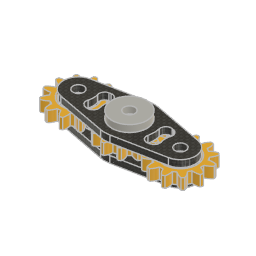
Gear fidget spinner thingy (Autodesk Fusion 360 design; units mm, degrees)
Autodesk Fusion 360 part; units mm, degrees
sketch "Sketch1" plane through (0, 0, 0) normal (0, 0, 1) x (1, 0, 0)
  circle A0 centre (0, 0) radius 12
  line L0 (0, 0) -> (-37, 0) construction
  line L1 (0, 0) -> (37, 0) construction
  line L2 (-37, 0) -> (-37, 25) construction
  line L3 (-37, 0) -> (-37, -25) construction
  circle A1 centre (37, 0) radius 4
  circle A2 centre (-37, 0) radius 4
  line L4 (-3.4054, 17.6749) -> (-39.0811, 10.8013)
  line L5 (3.4054, 17.6749) -> (39.0811, 10.8013)
  line L6 (-3.4054, -17.6749) -> (-39.0811, -10.8013)
  arc A3 (-37, 11) -> (-37, -11) centre (-37, 0) ccw
  arc A4 (38.8507, -10.8432) -> (39.0811, 10.8013) centre (37, 0) ccw
  arc A5 (3.4054, 17.6749) -> (-3.4054, 17.6749) centre (0, 0) ccw
  arc A6 (-3.4054, -17.6749) -> (3.4054, -17.6749) centre (0, 0) ccw
  line L7 (18, 0) -> (26, 0) construction
  line L8 (18, 0) -> (22, 0) construction
  line L9 (-26, 0) -> (-18, 0) construction
  line L10 (-26, 0) -> (-22, 0) construction
  line L11 (-22, 0) -> (-22, 14) construction
  line L12 (-22, 14) -> (-22, -14.0923) construction
  line L13 (22, 0) -> (22, 14.0923) construction
  line L14 (22, 0) -> (22, -14.0923) construction
  line L15 (24.9994, 13.5145) -> (24.0534, 8.6047) construction
  line L16 (38.8512, -10.8456) -> (37.9053, -5.9359) construction
  line L17 (-22, -14.0923) -> (-21.9955, -14.0932) construction
  line L18 (-22, -14.0923) -> (-21.0541, -9.1826) construction
  line L19 (22.1718, 8.9673) -> (23.5375, 8.7041)
  line L20 (23.5375, -8.7041) -> (22.1718, -8.9673)
  line L21 (-22.1718, 8.9673) -> (-23.5375, 8.7041)
  line L22 (39.0811, -10.8013) -> (37, -11.2023)
  line L23 (38.8512, -10.8456) -> (3.4054, -17.6749)
  arc A7 (26.5726, 3.5027) -> (26.5726, -3.5027) centre (37, 0) ccw
  arc A8 (39.0811, -10.8013) -> (39.0811, 10.8013) centre (37, 0) ccw
  arc A9 (17.5214, -4.1232) -> (17.5214, 4.1232) centre (0, 0) ccw
  arc A10 (3.4054, 17.6749) -> (-3.4054, 17.6749) centre (0, 0) ccw
  arc A11 (-17.5214, 4.1232) -> (-17.5214, -4.1232) centre (0, 0) ccw
  arc A12 (-3.4054, -17.6749) -> (3.4054, -17.6749) centre (0, 0) ccw
  line L24 (-22.1718, -8.9673) -> (-23.5375, -8.7041)
  arc A13 (-26.5726, -3.5027) -> (-26.5726, 3.5027) centre (-37, 0) ccw
  arc A14 (-37, 11) -> (-37, -11) centre (-37, 0) ccw
  arc A15 (-17.5214, 4.1232) -> (-22.1718, 8.9673) centre (-21.415, 5.0395) ccw
  arc A16 (-23.5375, 8.7041) -> (-26.5726, 3.5027) centre (-22.7808, 4.7764) ccw
  arc A17 (-26.5726, -3.5027) -> (-23.5375, -8.7041) centre (-22.7808, -4.7764) ccw
  arc A18 (-22.1718, -8.9673) -> (-17.5214, -4.1232) centre (-21.415, -5.0395) ccw
  arc A19 (22.1718, 8.9673) -> (17.5214, 4.1232) centre (21.415, 5.0395) ccw
  arc A20 (26.5726, 3.5027) -> (23.5375, 8.7041) centre (22.7808, 4.7764) ccw
  arc A21 (23.5375, -8.7041) -> (26.5726, -3.5027) centre (22.7808, -4.7764) ccw
  arc A22 (17.5214, -4.1232) -> (22.1718, -8.9673) centre (21.415, -5.0395) ccw
  dimension "d1" = 24
  dimension "d2" = 36
  dimension "d3" = 37
  dimension "d4" = 37
  dimension "d5" = 8
  dimension "d6" = 22
  dimension "d7" = 8
  dimension "d8" = 22
  dimension "d9" = 36
  dimension "d10" = 22
  dimension "d11" = 22
  dimension "d12" = 5
  dimension "d13" = 5
  dimension "d14" = 5
  dimension "d17" = 4
  dimension "d18" = 4
  constraint coincident A0.centre L0.start
  constraint concentric A0 A5
  constraint horizontal L0
  constraint parallel L0 L1
  constraint perpendicular L0 L2
  constraint perpendicular L0 L3
  constraint coincident L1.end A1.centre
  constraint concentric A1 A4
  constraint coincident L0.end L2.start
  constraint concentric A2 A3
  constraint coincident L4.end A3
  constraint tangent L4 A3
  constraint tangent L4 A5
  constraint tangent L5 A4
  constraint tangent L5 A5
  constraint coincident L22.start A4
  constraint tangent A5 L22
  constraint coincident L6.start A5
  constraint coincident L6.end A3
  constraint tangent L6 A3
  constraint tangent L6 A5
  constraint tangent A4 L22
  constraint coincident L2 A3.start
  constraint coincident L3 A3.end
  constraint concentric A5 A6
  constraint concentric A0 A9
  constraint concentric A1 A7
  constraint coincident L1 L7.start
  constraint coincident L7.start A9
  constraint coincident L7.end A7
  constraint coincident L1 L7.end
  constraint midpoint L7 L8.end
  constraint concentric A2 A13
  constraint coincident L9.start A13
  constraint coincident L0 L9.start
  constraint coincident L0 L9.end
  constraint coincident L9.end A9
  constraint midpoint L9 L10.end
  constraint perpendicular L10 L11
  constraint coincident L6 L12.end
  constraint perpendicular L10 L12
  constraint coincident L5 L13.end
  constraint perpendicular L7 L13
  constraint coincident L14.end L22
  constraint perpendicular L1 L14
  constraint coincident L5 L15.start
  constraint perpendicular L5 L15
  constraint coincident L16.start L22
  constraint perpendicular L16 L22
  constraint coincident L6 L17.end
  constraint perpendicular L17 L18
  constraint collinear L22 L23
  constraint concentric A7 A8
  constraint concentric A9 A10
  constraint concentric A10 A11
  constraint concentric A11 A12
  constraint concentric A13 A14
  constraint tangent A11 A15
  constraint tangent L21 A15
  constraint tangent L21 A16
  constraint tangent A13 A16
  constraint equal A15 A16
  constraint tangent A13 A17
  constraint tangent L24 A17
  constraint equal A15 A17
  constraint tangent L24 A18
  constraint tangent A11 A18
  constraint equal A15 A18
  constraint tangent A9 A19
  constraint tangent L19 A19
  constraint tangent L19 A20
  constraint tangent A7 A20
  constraint equal A19 A20
  constraint tangent A7 A21
  constraint tangent L20 A21
  constraint equal A19 A21
  constraint tangent L20 A22
  constraint tangent A9 A22
  constraint equal A19 A22
  constraint tangent L23 A8
  constraint coincident L16 A4.start
  measures "d1" diameter of A0
  measures "d2" diameter of A5
  measures "d3" distance of A0.centre L0.end
  measures "d4" distance of A0.centre L1.end
  measures "d5" diameter of A1
  measures "d6" diameter of A4
  measures "d7" diameter of A2
  measures "d8" diameter of A3
  measures "d9" diameter of A9
  measures "d10" diameter of A7
  measures "d11" diameter of A13
  measures "d12" distance of L15.start L15.end
  measures "d13" distance of L16.start L16.end
  measures "d14" distance of L12.end L18.end
  measures "d17" radius of A15
  measures "d18" radius of A19
extrude "Extrude1" add sketch "Sketch1" along normal blind 5 makes body 1
copy_body "CopyPasteBodies1" bodies 1 makes body 2
move_body "Move1" bodies 2 to x (1, 0, 0) y (0, 1, 0) z (0, 0, 1) at (0, 0, 13)
sketch "Sketch2" plane through (0, 0, 0) normal (0, 0, 1) x (1, 0, 0)
  circle A0 centre (0, 50) radius 12
  line L0 (0, 50) -> (0, 50.4627) construction
  line L1 (0, 70) -> (-1, 70)
  line L2 (0, 70) -> (1, 70)
  line L3 (-10, 67.3205) -> (-9.134, 67.8205)
  line L4 (-10, 67.3205) -> (-10.866, 66.8205)
  line L5 (-17.7256, 59.2984) -> (-16.8205, 60.866)
  line L6 (-17.3205, 60) -> (-17.8205, 59.134)
  line L7 (-20, 50) -> (-20, 51)
  line L8 (-20, 50) -> (-20, 49)
  line L9 (-17.3205, 40) -> (-17.8205, 40.866)
  line L10 (-17.3205, 40) -> (-16.8205, 39.134)
  line L11 (-10, 32.6795) -> (-10.866, 33.1795)
  line L12 (-10, 32.6795) -> (-9.134, 32.1795)
  line L13 (0, 30) -> (-1, 30)
  line L14 (0, 30) -> (1, 30)
  line L15 (10, 32.6795) -> (9.134, 32.1795)
  line L16 (10, 32.6795) -> (10.866, 33.1795)
  line L17 (17.3205, 40) -> (16.8205, 39.134)
  line L18 (17.3205, 40) -> (17.8205, 40.866)
  line L19 (20, 50) -> (20, 49)
  line L20 (20, 50) -> (20, 51)
  line L21 (17.3205, 60) -> (17.8205, 59.134)
  line L22 (17.3205, 60) -> (16.8205, 60.866)
  line L23 (10, 67.3205) -> (10.866, 66.8205)
  line L24 (10, 67.3205) -> (9.134, 67.8205)
  arc A1 (-17.7256, 59.2984) -> (-17.6928, 58.9935) centre (-17.5004, 59.1684) ccw
  line L25 (0, 0) -> (0, 30)
  line L26 (0, 70) -> (0, 75)
  arc A2 (-1, 70) -> (-2.675, 64.7596) centre (7.824, 64.2917) ccw
  arc A3 (2.675, 64.7596) -> (1, 70) centre (-9.0903, 63.8869) ccw
  arc A4 (-5.0632, 64.1196) -> (-9.134, 67.8205) centre (-14.8159, 57.4813) ccw
  arc A5 (-10.866, 66.8205) -> (-9.6964, 61.4446) centre (-0.37, 66.289) ccw
  line L27 (-10, 67.3205) -> (-9.134, 67.8205)
  line L28 (-10, 67.3205) -> (-10.866, 66.8205)
  arc A6 (-11.4446, 59.6964) -> (-16.8205, 60.866) centre (-16.5716, 49.0711) ccw
  arc A7 (-17.8205, 59.134) -> (-14.1196, 55.0632) centre (-8.4649, 63.9216) ccw
  line L29 (-17.3205, 60) -> (-16.8205, 60.866)
  line L30 (-17.3205, 60) -> (-17.8205, 59.134)
  arc A8 (-14.7596, 52.675) -> (-20, 51) centre (-13.8869, 40.9097) ccw
  arc A9 (-20, 49) -> (-14.7596, 47.325) centre (-14.2917, 57.824) ccw
  line L31 (-20, 50) -> (-20, 51)
  line L32 (-20, 50) -> (-20, 49)
  arc A10 (-14.1196, 44.9368) -> (-17.8205, 40.866) centre (-7.4813, 35.1841) ccw
  arc A11 (-16.8205, 39.134) -> (-11.4446, 40.3036) centre (-16.289, 49.63) ccw
  line L33 (-17.3205, 40) -> (-17.8205, 40.866)
  line L34 (-17.3205, 40) -> (-16.8205, 39.134)
  arc A12 (-9.6964, 38.5554) -> (-10.866, 33.1795) centre (0.9289, 33.4284) ccw
  arc A13 (-9.134, 32.1795) -> (-5.0632, 35.8804) centre (-13.9216, 41.5351) ccw
  line L35 (-10, 32.6795) -> (-10.866, 33.1795)
  line L36 (-10, 32.6795) -> (-9.134, 32.1795)
  arc A14 (-2.675, 35.2404) -> (-1, 30) centre (9.0903, 36.1131) ccw
  arc A15 (1, 30) -> (2.675, 35.2404) centre (-7.824, 35.7083) ccw
  line L37 (0, 30) -> (-1, 30)
  line L38 (0, 30) -> (1, 30)
  arc A16 (5.0632, 35.8804) -> (9.134, 32.1795) centre (14.8159, 42.5187) ccw
  arc A17 (10.866, 33.1795) -> (9.6964, 38.5554) centre (0.37, 33.711) ccw
  line L39 (10, 32.6795) -> (9.134, 32.1795)
  line L40 (10, 32.6795) -> (10.866, 33.1795)
  arc A18 (11.4446, 40.3036) -> (16.8205, 39.134) centre (16.5716, 50.9289) ccw
  arc A19 (17.8205, 40.866) -> (14.1196, 44.9368) centre (8.4649, 36.0784) ccw
  line L41 (17.3205, 40) -> (16.8205, 39.134)
  line L42 (17.3205, 40) -> (17.8205, 40.866)
  arc A20 (14.7596, 47.325) -> (20, 49) centre (13.8869, 59.0903) ccw
  arc A21 (20, 51) -> (14.7596, 52.675) centre (14.2917, 42.176) ccw
  line L43 (20, 50) -> (20, 49)
  line L44 (20, 50) -> (20, 51)
  arc A22 (14.1196, 55.0632) -> (17.8205, 59.134) centre (7.4813, 64.8159) ccw
  arc A23 (16.8205, 60.866) -> (11.4446, 59.6964) centre (16.289, 50.37) ccw
  line L45 (17.3205, 60) -> (17.8205, 59.134)
  line L46 (17.3205, 60) -> (16.8205, 60.866)
  arc A24 (9.6964, 61.4446) -> (10.866, 66.8205) centre (-0.9289, 66.5716) ccw
  arc A25 (9.134, 67.8205) -> (5.0632, 64.1196) centre (13.9216, 58.4649) ccw
  line L47 (10, 67.3205) -> (10.866, 66.8205)
  line L48 (10, 67.3205) -> (9.134, 67.8205)
  arc A26 (-2.675, 64.7596) -> (-5.0632, 64.1196) centre (0, 50) ccw
  arc A27 (5.0632, 64.1196) -> (2.675, 64.7596) centre (0, 50) ccw
  arc A28 (-9.6964, 61.4446) -> (-11.4446, 59.6964) centre (0, 50) ccw
  arc A29 (-14.1196, 55.0632) -> (-14.7596, 52.675) centre (0, 50) ccw
  arc A30 (2.675, 35.2404) -> (5.0632, 35.8804) centre (0, 50) ccw
  arc A31 (-5.0632, 35.8804) -> (-2.675, 35.2404) centre (0, 50) ccw
  arc A32 (-14.7596, 47.325) -> (-14.1196, 44.9368) centre (0, 50) ccw
  arc A33 (-11.4446, 40.3036) -> (-9.6964, 38.5554) centre (0, 50) ccw
  arc A34 (11.4446, 59.6964) -> (9.6964, 61.4446) centre (0, 50) ccw
  arc A35 (14.7596, 52.675) -> (14.1196, 55.0632) centre (0, 50) ccw
  arc A36 (9.6964, 38.5554) -> (11.4446, 40.3036) centre (0, 50) ccw
  arc A37 (14.1196, 44.9368) -> (14.7596, 47.325) centre (0, 50) ccw
  dimension "d21" = 24
  dimension "d22" = 30
  dimension "d25" = 20
  dimension "d26" = 1
  dimension "d27" = 1
  dimension "d30" = 0.26
  dimension "d32" = 360
  constraint coincident L25.start origin
  constraint vertical L25
  constraint coincident A0.centre L25
  constraint concentric A0 A26
  constraint coincident A0.centre L0.start
  constraint coincident L0.end L25
  constraint perpendicular L1 L25
  constraint perpendicular L2 L25
  constraint coincident L6.start L5
  constraint tangent L5 A1
  constraint collinear L25 L26
  constraint concentric A26 A28
  constraint concentric A27 A28
  constraint concentric A28 A32
  constraint concentric A28 A29
  constraint concentric A32 A36
  constraint concentric A30 A32
  constraint concentric A31 A32
  constraint concentric A32 A33
  constraint concentric A34 A36
  constraint concentric A35 A36
  constraint concentric A36 A37
  measures "d21" diameter of A0
  measures "d22" diameter of A26
  measures "d25" distance of A0.centre L1.start
  measures "d26" distance of L1.start L1.end
  measures "d27" distance of L1.start L2.end
  measures "d30" radius of A1
extrude "Extrude2" add sketch "Sketch2" along normal blind 8 separate body makes body 3
sketch "Sketch3" plane through (0, 0, 0) normal (0, 0, 1) x (1, 0, 0)
  circle A0 centre (0, 125) radius 12
  line L0 (-1, 145) -> (1, 145) construction
  line L1 (0, 145) -> (-1, 145)
  line L2 (0, 145) -> (1, 145)
  arc A1 (-1, 145) -> (-2.675, 139.7596) centre (8.0445, 139.2212) ccw
  arc A2 (2.675, 139.7596) -> (1, 145) centre (-8.4873, 139.0797) ccw
  line L3 (2.675, 145) -> (2.675, 145.0175) construction
  line L4 (2.675, 145.0175) -> (2.675, 145) construction
  line L5 (-1, 145) -> (1, 145)
  arc A3 (-5.0632, 139.1196) -> (-9.134, 142.8205) centre (-14.3901, 132.9497) ccw
  arc A4 (-10.866, 141.8205) -> (-9.6964, 136.4446) centre (-0.1439, 141.3382) ccw
  line L6 (-10.866, 141.8205) -> (-9.134, 142.8205) construction
  arc A5 (-11.4446, 134.6964) -> (-16.8205, 135.866) centre (-16.437, 124.6896) ccw
  arc A6 (-17.8205, 134.134) -> (-14.1196, 130.0632) centre (-8.2937, 139.0773) ccw
  line L7 (-17.8205, 134.134) -> (-16.8205, 135.866) construction
  arc A7 (-14.7596, 127.675) -> (-20, 126) centre (-14.0797, 116.5127) ccw
  arc A8 (-20, 124) -> (-14.7596, 122.325) centre (-14.2212, 133.0445) ccw
  line L8 (-20, 124) -> (-20, 126) construction
  arc A9 (-14.1196, 119.9368) -> (-17.8205, 115.866) centre (-7.9497, 110.6099) ccw
  arc A10 (-16.8205, 114.134) -> (-11.4446, 115.3036) centre (-16.3382, 124.8561) ccw
  line L9 (-16.8205, 114.134) -> (-17.8205, 115.866) construction
  arc A11 (-9.6964, 113.5554) -> (-10.866, 108.1795) centre (0.3104, 108.563) ccw
  arc A12 (-9.134, 107.1795) -> (-5.0632, 110.8804) centre (-14.0773, 116.7063) ccw
  line L10 (-9.134, 107.1795) -> (-10.866, 108.1795) construction
  arc A13 (-2.675, 110.2404) -> (-1, 105) centre (8.4873, 110.9203) ccw
  arc A14 (1, 105) -> (2.675, 110.2404) centre (-8.0445, 110.7788) ccw
  line L11 (1, 105) -> (-1, 105) construction
  arc A15 (5.0632, 110.8804) -> (9.134, 107.1795) centre (14.3901, 117.0503) ccw
  arc A16 (10.866, 108.1795) -> (9.6964, 113.5554) centre (0.1439, 108.6618) ccw
  line L12 (10.866, 108.1795) -> (9.134, 107.1795) construction
  arc A17 (11.4446, 115.3036) -> (16.8205, 114.134) centre (16.437, 125.3104) ccw
  arc A18 (17.8205, 115.866) -> (14.1196, 119.9368) centre (8.2937, 110.9227) ccw
  line L13 (17.8205, 115.866) -> (16.8205, 114.134) construction
  arc A19 (14.7596, 122.325) -> (20, 124) centre (14.0797, 133.4873) ccw
  arc A20 (20, 126) -> (14.7596, 127.675) centre (14.2212, 116.9555) ccw
  line L14 (20, 126) -> (20, 124) construction
  arc A21 (14.1196, 130.0632) -> (17.8205, 134.134) centre (7.9497, 139.3901) ccw
  arc A22 (16.8205, 135.866) -> (11.4446, 134.6964) centre (16.3382, 125.1439) ccw
  line L15 (16.8205, 135.866) -> (17.8205, 134.134) construction
  arc A23 (9.6964, 136.4446) -> (10.866, 141.8205) centre (-0.3104, 141.437) ccw
  arc A24 (9.134, 142.8205) -> (5.0632, 139.1196) centre (14.0773, 133.2937) ccw
  line L16 (9.134, 142.8205) -> (10.866, 141.8205) construction
  arc A25 (-9.6964, 136.4446) -> (-11.4446, 134.6964) centre (0, 125) ccw
  arc A26 (-14.1196, 130.0632) -> (-14.7596, 127.675) centre (0, 125) ccw
  arc A27 (-14.7596, 122.325) -> (-14.1196, 119.9368) centre (0, 125) ccw
  arc A28 (-11.4446, 115.3036) -> (-9.6964, 113.5554) centre (0, 125) ccw
  arc A29 (-5.0632, 110.8804) -> (-2.675, 110.2404) centre (0, 125) ccw
  arc A30 (2.675, 110.2404) -> (5.0632, 110.8804) centre (0, 125) ccw
  arc A31 (9.6964, 113.5554) -> (11.4446, 115.3036) centre (0, 125) ccw
  arc A32 (14.1196, 119.9368) -> (14.7596, 122.325) centre (0, 125) ccw
  arc A33 (14.7596, 127.675) -> (14.1196, 130.0632) centre (0, 125) ccw
  arc A34 (11.4446, 134.6964) -> (9.6964, 136.4446) centre (0, 125) ccw
  arc A35 (5.0632, 139.1196) -> (2.675, 139.7596) centre (0, 125) ccw
  arc A36 (-2.675, 139.7596) -> (-5.0632, 139.1196) centre (0, 125) ccw
  line L17 (-10.866, 141.8205) -> (-9.134, 142.8205)
  line L18 (-1, 145) -> (1, 145)
  line L19 (9.134, 142.8205) -> (10.866, 141.8205)
  line L20 (16.8205, 135.866) -> (17.8205, 134.134)
  line L21 (20, 126) -> (20, 124)
  line L22 (17.8205, 115.866) -> (16.8205, 114.134)
  line L23 (10.866, 108.1795) -> (9.134, 107.1795)
  line L24 (1, 105) -> (-1, 105)
  line L25 (-9.134, 107.1795) -> (-10.866, 108.1795)
  line L26 (-16.8205, 114.134) -> (-17.8205, 115.866)
  line L27 (-20, 124) -> (-20, 126)
  line L28 (-17.8205, 134.134) -> (-16.8205, 135.866)
  dimension "d35" = 24
  dimension "d36" = 30
  dimension "d39" = 20
  dimension "d40" = 1
  dimension "d41" = 1
  dimension "d43" = 360
  constraint concentric A0 A25
  constraint horizontal L0
  constraint coincident A1.end A25
  constraint coincident A2.start L4
  constraint coincident A2.start A25
  constraint concentric A25 A26
  constraint concentric A26 A27
  constraint concentric A27 A28
  constraint concentric A28 A29
  constraint concentric A29 A30
  constraint concentric A30 A31
  constraint concentric A31 A32
  constraint concentric A32 A33
  constraint concentric A33 A34
  constraint concentric A34 A35
  constraint concentric A35 A36
  measures "d35" diameter of A0
  measures "d36" diameter of A25
  measures "d39" distance of A0.centre L1.start
  measures "d40" distance of L1.start L0.start
  measures "d41" distance of L1.start L0.end
extrude "Extrude3" add sketch "Sketch3" along normal blind 8 separate body makes body 4
sketch "Sketch4" plane through (0, 0, 0) normal (0, 0, 1) x (1, 0, 0)
  circle A0 centre (150, 0) radius 4
  line L0 (150, 15) -> (150, -15) construction
  line L1 (135, 0) -> (165, 0) construction
  line L2 (150, 0) -> (152.675, 0) construction
  line L3 (150, 0) -> (147.325, 0) construction
  line L4 (147.325, 0) -> (147.325, 14.7596) construction
  line L5 (147.325, 0) -> (147.325, -14.7596) construction
  line L6 (152.675, 0) -> (152.675, 14.7596) construction
  line L7 (152.675, 0) -> (152.675, -14.7596) construction
  line L8 (150, 0) -> (150, 4) construction
  line L9 (150, 20) -> (149, 20)
  line L10 (150, 20) -> (151, 20)
  arc A1 (149, 20) -> (147.325, 14.7596) centre (158.0807, 14.2096) ccw
  arc A2 (152.675, 14.7596) -> (151, 20) centre (142.0972, 14.2665) ccw
  line L11 (140, 17.3205) -> (139.134, 16.8205)
  line L12 (140, 17.3205) -> (140.866, 17.8205)
  arc A3 (144.9368, 14.1196) -> (140.866, 17.8205) centre (136.0228, 8.4038) ccw
  arc A4 (139.134, 16.8205) -> (140.3036, 11.4446) centre (149.8933, 16.3463) ccw
  line L13 (132.6795, 10) -> (132.1795, 9.134)
  line L14 (132.6795, 10) -> (133.1795, 10.866)
  arc A5 (138.5554, 9.6964) -> (133.1795, 10.866) centre (133.6935, 0.2893) ccw
  arc A6 (132.1795, 9.134) -> (135.8804, 5.0632) centre (141.7345, 14.1029) ccw
  line L15 (130, 0) -> (130, -1)
  line L16 (130, 0) -> (130, 1)
  arc A7 (135.2404, 2.675) -> (130, 1) centre (135.7335, -7.9028) ccw
  arc A8 (130, -1) -> (135.2404, -2.675) centre (135.7904, 8.0807) ccw
  line L17 (132.6795, -10) -> (133.1795, -10.866)
  line L18 (132.6795, -10) -> (132.1795, -9.134)
  arc A9 (135.8804, -5.0632) -> (132.1795, -9.134) centre (141.5962, -13.9772) ccw
  arc A10 (133.1795, -10.866) -> (138.5554, -9.6964) centre (133.6537, -0.1067) ccw
  line L19 (140, -17.3205) -> (140.866, -17.8205)
  line L20 (140, -17.3205) -> (139.134, -16.8205)
  arc A11 (140.3036, -11.4446) -> (139.134, -16.8205) centre (149.7107, -16.3065) ccw
  arc A12 (140.866, -17.8205) -> (144.9368, -14.1196) centre (135.8971, -8.2655) ccw
  line L21 (150, -20) -> (151, -20)
  line L22 (150, -20) -> (149, -20)
  arc A13 (147.325, -14.7596) -> (149, -20) centre (157.9028, -14.2665) ccw
  arc A14 (151, -20) -> (152.675, -14.7596) centre (141.9193, -14.2096) ccw
  line L23 (160, -17.3205) -> (160.866, -16.8205)
  line L24 (160, -17.3205) -> (159.134, -17.8205)
  arc A15 (155.0632, -14.1196) -> (159.134, -17.8205) centre (163.9772, -8.4038) ccw
  arc A16 (160.866, -16.8205) -> (159.6964, -11.4446) centre (150.1067, -16.3463) ccw
  line L25 (167.3205, -10) -> (167.8205, -9.134)
  line L26 (167.3205, -10) -> (166.8205, -10.866)
  arc A17 (161.4446, -9.6964) -> (166.8205, -10.866) centre (166.3065, -0.2893) ccw
  arc A18 (167.8205, -9.134) -> (164.1196, -5.0632) centre (158.2655, -14.1029) ccw
  line L27 (170, 0) -> (170, 1)
  line L28 (170, 0) -> (170, -1)
  arc A19 (164.7596, -2.675) -> (170, -1) centre (164.2665, 7.9028) ccw
  arc A20 (170, 1) -> (164.7596, 2.675) centre (164.2096, -8.0807) ccw
  line L29 (167.3205, 10) -> (166.8205, 10.866)
  line L30 (167.3205, 10) -> (167.8205, 9.134)
  arc A21 (164.1196, 5.0632) -> (167.8205, 9.134) centre (158.4038, 13.9772) ccw
  arc A22 (166.8205, 10.866) -> (161.4446, 9.6964) centre (166.3463, 0.1067) ccw
  line L31 (160, 17.3205) -> (159.134, 17.8205)
  line L32 (160, 17.3205) -> (160.866, 16.8205)
  arc A23 (159.6964, 11.4446) -> (160.866, 16.8205) centre (150.2893, 16.3065) ccw
  arc A24 (159.134, 17.8205) -> (155.0632, 14.1196) centre (164.1029, 8.2655) ccw
  arc A25 (147.325, 14.7596) -> (144.9368, 14.1196) centre (150, 0) ccw
  arc A26 (155.0632, 14.1196) -> (152.675, 14.7596) centre (150, 0) ccw
  arc A27 (161.4446, 9.6964) -> (159.6964, 11.4446) centre (150, 0) ccw
  arc A28 (164.7596, 2.675) -> (164.1196, 5.0632) centre (150, 0) ccw
  arc A29 (164.1196, -5.0632) -> (164.7596, -2.675) centre (150, 0) ccw
  arc A30 (159.6964, -11.4446) -> (161.4446, -9.6964) centre (150, 0) ccw
  arc A31 (152.675, -14.7596) -> (155.0632, -14.1196) centre (150, 0) ccw
  arc A32 (144.9368, -14.1196) -> (147.325, -14.7596) centre (150, 0) ccw
  arc A33 (138.5554, -9.6964) -> (140.3036, -11.4446) centre (150, 0) ccw
  arc A34 (135.2404, -2.675) -> (135.8804, -5.0632) centre (150, 0) ccw
  arc A35 (140.3036, 11.4446) -> (138.5554, 9.6964) centre (150, 0) ccw
  arc A36 (135.8804, 5.0632) -> (135.2404, 2.675) centre (150, 0) ccw
  dimension "d46" = 8
  dimension "d47" = 30
  dimension "d48" = 2.675
  dimension "d49" = 2.675
  dimension "d50" = 20
  dimension "d51" = 1
  dimension "d52" = 1
  dimension "d54" = 360
  constraint concentric A0 A25
  constraint coincident L0.end A25
  constraint vertical L0
  constraint coincident L1.start A25
  constraint coincident L1.end A25
  constraint perpendicular L0 L1
  constraint coincident A0.centre L2.start
  constraint perpendicular L0 L2
  constraint coincident L1 L3.end
  constraint perpendicular L0 L3
  constraint perpendicular L1 L4
  constraint coincident L5.end A25
  constraint perpendicular L3 L5
  constraint perpendicular L1 L6
  constraint coincident L7.end A25
  constraint perpendicular L1 L7
  constraint perpendicular L3 L8
  constraint perpendicular L8 L9
  constraint perpendicular L8 L10
  constraint coincident A0 L8.end
  constraint concentric A25 A35
  constraint concentric A26 A35
  constraint concentric A27 A35
  constraint concentric A28 A35
  constraint concentric A29 A35
  constraint concentric A30 A35
  constraint concentric A31 A35
  constraint concentric A32 A35
  constraint concentric A33 A35
  constraint concentric A34 A35
  constraint concentric A35 A36
  measures "d46" diameter of A0
  measures "d47" diameter of A25
  measures "d48" distance of A0.centre L2.end
  measures "d49" distance of A0.centre L3.end
  measures "d50" distance of A0.centre L9.start
  measures "d51" distance of L9.start L9.end
  measures "d52" distance of L9.start L10.end
extrude "Extrude4" add sketch "Sketch4" along normal blind 8 separate body makes body 5
copy_body "Body->Comp1" bodies 1 removing the originals makes body 6 in component "bottom cover"
copy_body "Body->Comp2" bodies 2 removing the originals makes body 7 in component "top cover"
copy_body "Body->Comp3" bodies 3 removing the originals makes body 8 in component "gear 1"
copy_body "Body->Comp4" bodies 4 removing the originals makes body 9 in component "gear 2"
copy_body "Body->Comp5" bodies 5 removing the originals makes body 10 in component "gear 3"
sketch "Sketch6" plane through (0, 0, 0) normal (0, 1, 0) x (1, 0, 0)
  circle A0 centre (0, -40) radius 4
  circle A1 centre (0, -40) radius 13
  circle A2 centre (0, -40) radius 3.75
  circle A3 centre (0, -40) radius 12.75
  dimension "d69" = 8
  dimension "d70" = 26
  dimension "d71" = 7.5
  dimension "d72" = 25.5
  constraint concentric A0 A1
  constraint concentric A0 A2
  constraint concentric A2 A3
  measures "d69" diameter of A0
  measures "d70" diameter of A1
  measures "d71" diameter of A2
  measures "d72" diameter of A3
extrude "Extrude5" add sketch "Sketch6" along normal blind 5 separate body contours A3 makes body 11
move_body "Move2" bodies 11 to x (0.996195, -0.087156, 0) y (0, 0, -1) z (0.087156, 0.996195, 0) at (-3.4862, -39.8478, 40)
copy_body "Body->Comp6" bodies 11 removing the originals makes body 12 in component "top component"
component "bottom cover" placed x (1, 0, 0) y (0, 1, 0) z (0, 0, 1) at (0, 0, 0)
component "top cover" placed x (0.999989, 0.004655, 0) y (-0.004655, 0.999989, 0) z (0, 0, 1) at (0, 0, 0)
component "gear 1" placed x (0.97802, 0.208509, 0) y (-0.208509, 0.97802, 0) z (0, 0, 1) at (-26.5741, -49.0733, 5)
component "gear 2" placed x (0.97778, 0.209635, 0) y (-0.209635, 0.97778, 0) z (0, 0, 1) at (63.204, -122.0502, 5)
component "gear 3" placed x (0.999989, 0.004655, 0) y (-0.004655, 0.999989, 0) z (0, 0, 1) at (-149.9984, -0.6983, 5)
component "top component" placed x (0.75687, 0.653566, 0) y (-0.653566, 0.75687, 0) z (0, 0, 1) at (0, 0, -17)
